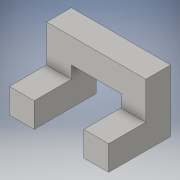
# Autodesk Inventor part: Figure 7_27_5
Saved by Autodesk Inventor 2016 (Build 200138000, 138)
## iProperties
Created: 2016-07-18
Part Number: Figure 7_27_5
Material: Generic
Document SubType Name: Modeling
Designer: cfkguest
Density: 1 g/cm^3
Appearance: Default
Author: cfkguest
Autodesk Inventor part; units mm, degrees
ref_plane "YZ Plane" through (0, 0, 0) normal (1, 0, 0) x (0, 1, 0)
ref_plane "XZ Plane" through (0, 0, 0) normal (0, 1, 0) x (-1, 0, 0)
ref_plane "XY Plane" through (0, 0, 0) normal (0, 0, 1) x (1, 0, 0)
sketch "Sketch1" plane through (0, 0, 0) normal (0, 0, 1) x (1, 0, 0)
  line L0 (-27.1073, 14.808) -> (23.6927, 14.808)
  line L1 (23.6927, 14.808) -> (23.6927, -16.942)
  line L2 (23.6927, -16.942) -> (-27.1073, -16.942)
  line L3 (-27.1073, -16.942) -> (-27.1073, 14.808)
  point P0 (0, 0)
  dimension "d0" = 50.8
  dimension "d1" = 31.75
  constraints: 8 end point, 2 parallel, 1 horizontal, 1 perpendicular
  measures "d0" distance of L0.start L0.end
  measures "d1" distance of L2.end L0.start
extrude "Extrusion1" add sketch "Sketch1" along normal blind 31.75
sketch "Sketch2" plane through (0, 0, 31.75) normal (0, 0, 1) x (1, 0, 0)
  line L0 (-27.1073, -16.942) -> (23.6927, -16.942) projected
  line L1 (-14.4073, -16.942) -> (10.9927, -16.942)
  line L2 (10.9927, -16.942) -> (10.9927, 2.108)
  line L3 (10.9927, 2.108) -> (-14.4073, 2.108)
  line L4 (-14.4073, 2.108) -> (-14.4073, -16.942)
  line L5 (-27.1073, 14.808) -> (-27.1073, -16.942) projected
  line L6 (23.6927, -16.942) -> (23.6927, 14.808) projected
  point P0 (0, 0)
  dimension "d4" = 12.7
  dimension "d5" = 12.7
  dimension "d6" = 19.05
  constraints: 8 end point, 2 parallel, 1 horizontal, 1 perpendicular, 1 point on line
  measures "d4" distance between parallel lines of L5 L4
  measures "d5" distance between parallel lines of L6 L2
  measures "d6" distance of L3.end L1.start
extrude "Extrusion2" cut sketch "Sketch2" against normal blind 31.75
sketch "Sketch3" plane through (23.6927, -16.942, 0) normal (1, 0, 0) x (0, 0, -1)
  line L0 (-31.75, 0) -> (-31.75, 31.75) projected
  line L1 (-31.75, 31.75) -> (-12.7, 31.75)
  line L2 (-12.7, 31.75) -> (-12.7, 12.7)
  line L3 (-12.7, 12.7) -> (-31.75, 12.7)
  line L4 (-31.75, 12.7) -> (-31.75, 31.75)
  point P0 (0, 16.942)
  dimension "d9" = 19.05
  dimension "d10" = 19.05
  constraints: 8 end point, 2 parallel, 1 horizontal, 1 perpendicular
  measures "d9" distance of L1.end L2.end
  measures "d10" distance of L2.end L3.end
extrude "Extrusion3" cut sketch "Sketch3" against normal blind 50.8
body "Solid1"
